Autodesk Fusion 360 part; units mm, degrees
(part 6 of 6)
extrude "Extrude3" cut sketch "Sketch2" along normal blind 1 contours L6 L7 L8 L9 L10 A2 | L11 L12 L13 L14 | L15 L16 L17 L18 L19 L20 | L21 L22 L23 L24 L25 A1 | L26 L27 L28 L29 | L30 L31 L32 L33 L34 A4 | L35 L36 L37 L38 L39 A3 | A0 | L40 L62 L64 L70 | L41 A7 L61 L63 L67 L73 | A5 L43 L48 L52 L55 L60 | A6 | L42 L46 L47 L54 L59 A8 | L44 L49 L53 L56 | L45 L50 L57 L66 L68 L71 | L51 L58 A9 L65 L69 L72 | L74 L96 L98 L104 | L75 A12 L95 L97 L101 L107 | A10 L77 L82 L86 L89 L94 | A11 | L76 L80 L81 L88 L93 A13 | L78 L83 L87 L90 | L79 L84 L91 L100 L102 L105 | L85 L92 A14 L99 L103 L106 | L108 L130 L132 L138 | L109 A17 L129 L131 L135 L141 | A15 L111 L116 L120 L123 L128 | A16 | L110 L114 L115 L122 L127 A18 | L112 L117 L121 L124 | L113 L118 L125 L134 L136 L139 | L119 L126 A19 L133 L137 L140 | L142 L164 L166 L172 | L143 A22 L163 L165 L169 L175 | A20 L145 L150 L154 L157 L162 | A21 | L144 L148 L149 L156 L161 A23 | L146 L151 L155 L158 | L147 L152 L159 L168 L170 L173 | L153 L160 A24 L167 L171 L174 | L176 L198 L200 L206 | L177 A27 L197 L199 L203 L209 | A25 L179 L184 L188 L191 L196 | A26 | L178 L182 L183 L190 L195 A28 | L180 L185 L189 L192 | L181 L186 L193 L202 L204 L207 | L187 L194 A29 L201 L205 L208 | L210 L232 L234 L240 | L211 A32 L231 L233 L237 L243 | A30 L213 L218 L222 L225 L230 | A31 | L212 L216 L217 L224 L229 A33 | L214 L219 L223 L226 | L215 L220 L227 L236 L238 L241 | L221 L228 A34 L235 L239 L242 | L244 L266 L268 L274 | L245 A37 L265 L267 L271 L277 | A35 L247 L252 L256 L259 L264 | A36 | L246 L250 L251 L258 L263 A38 | L248 L253 L257 L260 | L249 L254 L261 L270 L272 L275 | L255 L262 A39 L269 L273 L276 | L278 L300 L302 L308 | L279 A42 L299 L301 L305 L311 | A40 L281 L286 L290 L293 L298 | A41 | L280 L284 L285 L292 L297 A43 | L282 L287 L291 L294 | L283 L288 L295 L304 L306 L309 | L289 L296 A44 L303 L307 L310 | L312 L334 L336 L342 | L313 A47 L333 L335 L339 L345 | A45 L315 L320 L324 L327 L332 | A46 | L314 L318 L319 L326 L331 A48 | L316 L321 L325 L328 | L317 L322 L329 L338 L340 L343 | L323 L330 A49 L337 L341 L344 | L346 L368 L370 L376 | L347 A52 L367 L369 L373 L379 | A50 L349 L354 L358 L361 L366 | A51 | L348 L352 L353 L360 L365 A53 | L350 L355 L359 L362 | L351 L356 L363 L372 L374 L377 | L357 L364 A54 L371 L375 L378 | L380 L402 L404 L410 | L381 A57 L401 L403 L407 L413 | A55 L383 L388 L392 L395 L400 | A56 | L382 L386 L387 L394 L399 A58 | L384 L389 L393 L396 | L385 L390 L397 L406 L408 L411 | L391 L398 A59 L405 L409 L412 | L414 L436 L438 L444 | L415 A62 L435 L437 L441 L447 | A60 L417 L422 L426 L429 L434 | A61 | L416 L420 L421 L428 L433 A63 | L418 L423 L427 L430 | L419 L424 L431 L440 L442 L445 | L425 L432 A64 L439 L443 L446 | L448 L470 L472 L478 | L449 A67 L469 L471 L475 L481 | A65 L451 L456 L460 L463 L468 | A66 | L450 L454 L455 L462 L467 A68 | L452 L457 L461 L464 | L453 L458 L465 L474 L476 L479 | L459 L466 A69 L473 L477 L480 | L482 L504 L506 L512 | L483 A72 L503 L505 L509 L515 | A70 L485 L490 L494 L497 L502 | A71 | L484 L488 L489 L496 L501 A73 | L486 L491 L495 L498 | L487 L492 L499 L508 L510 L513 | L493 L500 A74 L507 L511 L514 | L516 L538 L540 L546 | L517 A77 L537 L539 L543 L549 | A75 L519 L524 L528 L531 L536 | A76 | L518 L522 L523 L530 L535 A78 | L520 L525 L529 L532 | L521 L526 L533 L542 L544 L547 | L527 L534 A79 L541 L545 L548 | L550 L572 L574 L580 | L551 A82 L571 L573 L577 L583 | A80 L553 L558 L562 L565 L570 | A81 | L552 L556 L557 L564 L569 A83 | L554 L559 L563 L566 | L555 L560 L567 L576 L578 L581 | L561 L568 A84 L575 L579 L582 | L584 L606 L608 L614 | L585 A87 L605 L607 L611 L617 | A85 L587 L592 L596 L599 L604 | A86 | L586 L590 L591 L598 L603 A88 | L588 L593 L597 L600 | L589 L594 L601 L610 L612 L615 | L595 L602 A89 L609 L613 L616 | L618 L640 L642 L648 | L619 A92 L639 L641 L645 L651 | A90 L621 L626 L630 L633 L638 | A91 | L620 L624 L625 L632 L637 A93 | L622 L627 L631 L634 | L623 L628 L635 L644 L646 L649 | L629 L636 A94 L643 L647 L650 | L652 L674 L676 L682 | L653 A97 L673 L675 L679 L685 | A95 L655 L660 L664 L667 L672 | A96 | L654 L658 L659 L666 L671 A98 | L656 L661 L665 L668 | L657 L662 L669 L678 L680 L683 | L663 L670 A99 L677 L681 L684 | L686 L708 L710 L716 | L687 A102 L707 L709 L713 L719 | A100 L689 L694 L698 L701 L706 | A101 | L688 L692 L693 L700 L705 A103 | L690 L695 L699 L702 | L691 L696 L703 L712 L714 L717 | L697 L704 A104 L711 L715 L718 | L720 L742 L744 L750 | L721 A107 L741 L743 L747 L753 | A105 L723 L728 L732 L735 L740 | A106 | L722 L726 L727 L734 L739 A108 | L724 L729 L733 L736 | L725 L730 L737 L746 L748 L751 | L731 L738 A109 L745 L749 L752 | L754 L776 L778 L784 | L755 A112 L775 L777 L781 L787 | A110 L757 L762 L766 L769 L774 | A111 | L756 L760 L761 L768 L773 A113 | L758 L763 L767 L770 | L759 L764 L771 L780 L782 L785 | L765 L772 A114 L779 L783 L786 | L788 L810 L812 L818 | L789 A117 L809 L811 L815 L821 | A115 L791 L796 L800 L803 L808 | A116 | L790 L794 L795 L802 L807 A118 | L792 L797 L801 L804 | L793 L798 L805 L814 L816 L819 | L799 L806 A119 L813 L817 L820 | L822 L844 L846 L852 | L823 A122 L843 L845 L849 L855 | A120 L825 L830 L834 L837 L842 | A121 | L824 L828 L829 L836 L841 A123 | L826 L831 L835 L838 | L827 L832 L839 L848 L850 L853 | L833 L840 A124 L847 L851 L854 | L856 L878 L880 L886 | L857 A127 L877 L879 L883 L889 | A125 L859 L864 L868 L871 L876 | A126 | L858 L862 L863 L870 L875 A128 | L860 L865 L869 L872 | L861 L866 L873 L882 L884 L887 | L867 L874 A129 L881 L885 L888 | L890 L912 L914 L920 | L891 A132 L911 L913 L917 L923 | A130 L893 L898 L902 L905 L910 | A131 | L892 L896 L897 L904 L909 A133 | L894 L899 L903 L906 | L895 L900 L907 L916 L918 L921 | L901 L908 A134 L915 L919 L922 | L924 L946 L948 L954 | L925 A137 L945 L947 L951 L957 | A135 L927 L932 L936 L939 L944 | A136 | L926 L930 L931 L938 L943 A138 | L928 L933 L937 L940 | L929 L934 L941 L950 L952 L955 | L935 L942 A139 L949 L953 L956 | L958 L980 L982 L988 | L959 A142 L979 L981 L985 L991 | A140 L961 L966 L970 L973 L978 | A141 | L960 L964 L965 L972 L977 A143 | L962 L967 L971 L974 | L963 L968 L975 L984 L986 L989 | L969 L976 A144 L983 L987 L990 | L992 L1014 L1016 L1022 | L993 A147 L1013 L1015 L1019 L1025 | A145 L995 L1000 L1004 L1007 L1012 | A146 | L994 L998 L999 L1006 L1011 A148 | L996 L1001 L1005 L1008 | L997 L1002 L1009 L1018 L1020 L1023 | L1003 L1010 A149 L1017 L1021 L1024 | L1026 L1048 L1050 L1056 | L1027 A152 L1047 L1049 L1053 L1059 | A150 L1029 L1034 L1038 L1041 L1046 | A151 | L1028 L1032 L1033 L1040 L1045 A153 | L1030 L1035 L1039 L1042 | L1031 L1036 L1043 L1052 L1054 L1057 | L1037 L1044 A154 L1051 L1055 L1058 | L1060 L1082 L1084 L1090 | L1061 A157 L1081 L1083 L1087 L1093 | A155 L1063 L1068 L1072 L1075 L1080 | A156 | L1062 L1066 L1067 L1074 L1079 A158 | L1064 L1069 L1073 L1076 | L1065 L1070 L1077 L1086 L1088 L1091 | L1071 L1078 A159 L1085 L1089 L1092
extrude "Extrude4" cut sketch "Sketch2" along normal blind 1 contours L1094 L1116 L1118 L1124 | L1095 A162 L1115 L1117 L1121 L1127 | A160 L1097 L1102 L1106 L1109 L1114 | A161 | L1096 L1100 L1101 L1108 L1113 A163 | L1098 L1103 L1107 L1110 | L1099 L1104 L1111 L1120 L1122 L1125 | L1105 L1112 A164 L1119 L1123 L1126 | L1128 L1150 L1152 L1158 | L1129 A167 L1149 L1151 L1155 L1161 | A165 L1131 L1136 L1140 L1143 L1148 | A166 | L1130 L1134 L1135 L1142 L1147 A168 | L1132 L1137 L1141 L1144 | L1133 L1138 L1145 L1154 L1156 L1159 | L1139 L1146 A169 L1153 L1157 L1160 | L1162 L1184 L1186 L1192 | L1163 A172 L1183 L1185 L1189 L1195 | A170 L1165 L1170 L1174 L1177 L1182 | A171 | L1164 L1168 L1169 L1176 L1181 A173 | L1166 L1171 L1175 L1178 | L1167 L1172 L1179 L1188 L1190 L1193 | L1173 L1180 A174 L1187 L1191 L1194 | L1196 L1218 L1220 L1226 | L1197 A177 L1217 L1219 L1223 L1229 | A175 L1199 L1204 L1208 L1211 L1216 | A176 | L1198 L1202 L1203 L1210 L1215 A178 | L1200 L1205 L1209 L1212 | L1201 L1206 L1213 L1222 L1224 L1227 | L1207 L1214 A179 L1221 L1225 L1228 | L1230 L1252 L1254 L1260 | L1231 A182 L1251 L1253 L1257 L1263 | A180 L1233 L1238 L1242 L1245 L1250 | A181 | L1232 L1236 L1237 L1244 L1249 A183 | L1234 L1239 L1243 L1246 | L1235 L1240 L1247 L1256 L1258 L1261 | L1241 L1248 A184 L1255 L1259 L1262 | L1264 L1286 L1288 L1294 | L1265 A187 L1285 L1287 L1291 L1297 | A185 L1267 L1272 L1276 L1279 L1284 | A186 | L1266 L1270 L1271 L1278 L1283 A188 | L1268 L1273 L1277 L1280 | L1269 L1274 L1281 L1290 L1292 L1295 | L1275 L1282 A189 L1289 L1293 L1296 | L1298 L1320 L1322 L1328 | L1299 A192 L1319 L1321 L1325 L1331 | A190 L1301 L1306 L1310 L1313 L1318 | A191 | L1300 L1304 L1305 L1312 L1317 A193 | L1302 L1307 L1311 L1314 | L1303 L1308 L1315 L1324 L1326 L1329 | L1309 L1316 A194 L1323 L1327 L1330 | L1332 L1354 L1356 L1362 | L1333 A197 L1353 L1355 L1359 L1365 | A195 L1335 L1340 L1344 L1347 L1352 | A196 | L1334 L1338 L1339 L1346 L1351 A198 | L1336 L1341 L1345 L1348 | L1337 L1342 L1349 L1358 L1360 L1363 | L1343 L1350 A199 L1357 L1361 L1364 | L1366 L1388 L1390 L1396 | L1367 A202 L1387 L1389 L1393 L1399 | A200 L1369 L1374 L1378 L1381 L1386 | A201 | L1368 L1372 L1373 L1380 L1385 A203 | L1370 L1375 L1379 L1382 | L1371 L1376 L1383 L1392 L1394 L1397 | L1377 L1384 A204 L1391 L1395 L1398 | L1400 L1422 L1424 L1430 | L1401 A207 L1421 L1423 L1427 L1433 | A205 L1403 L1408 L1412 L1415 L1420 | A206 | L1402 L1406 L1407 L1414 L1419 A208 | L1404 L1409 L1413 L1416 | L1405 L1410 L1417 L1426 L1428 L1431 | L1411 L1418 A209 L1425 L1429 L1432 | L1434 L1456 L1458 L1464 | L1435 A212 L1455 L1457 L1461 L1467 | A210 L1437 L1442 L1446 L1449 L1454 | A211 | L1436 L1440 L1441 L1448 L1453 A213 | L1438 L1443 L1447 L1450 | L1439 L1444 L1451 L1460 L1462 L1465 | L1445 L1452 A214 L1459 L1463 L1466 | L1468 L1490 L1492 L1498 | L1469 A217 L1489 L1491 L1495 L1501 | A215 L1471 L1476 L1480 L1483 L1488 | A216 | L1470 L1474 L1475 L1482 L1487 A218 | L1472 L1477 L1481 L1484 | L1473 L1478 L1485 L1494 L1496 L1499 | L1479 L1486 A219 L1493 L1497 L1500 | L1502 L1524 L1526 L1532 | L1503 A222 L1523 L1525 L1529 L1535 | A220 L1505 L1510 L1514 L1517 L1522 | A221 | L1504 L1508 L1509 L1516 L1521 A223 | L1506 L1511 L1515 L1518 | L1507 L1512 L1519 L1528 L1530 L1533 | L1513 L1520 A224 L1527 L1531 L1534 | L1536 L1558 L1560 L1566 | L1537 A227 L1557 L1559 L1563 L1569 | A225 L1539 L1544 L1548 L1551 L1556 | A226 | L1538 L1542 L1543 L1550 L1555 A228 | L1540 L1545 L1549 L1552 | L1541 L1546 L1553 L1562 L1564 L1567 | L1547 L1554 A229 L1561 L1565 L1568 | L1570 L1592 L1594 L1600 | L1571 A232 L1591 L1593 L1597 L1603 | A230 L1573 L1578 L1582 L1585 L1590 | A231 | L1572 L1576 L1577 L1584 L1589 A233 | L1574 L1579 L1583 L1586 | L1575 L1580 L1587 L1596 L1598 L1601 | L1581 L1588 A234 L1595 L1599 L1602 | L1604 L1626 L1628 L1634 | L1605 A237 L1625 L1627 L1631 L1637 | A235 L1607 L1612 L1616 L1619 L1624 | A236 | L1606 L1610 L1611 L1618 L1623 A238 | L1608 L1613 L1617 L1620 | L1609 L1614 L1621 L1630 L1632 L1635 | L1615 L1622 A239 L1629 L1633 L1636 | L1638 L1660 L1662 L1668 | L1639 A242 L1659 L1661 L1665 L1671 | A240 L1641 L1646 L1650 L1653 L1658 | A241 | L1640 L1644 L1645 L1652 L1657 A243 | L1642 L1647 L1651 L1654 | L1643 L1648 L1655 L1664 L1666 L1669 | L1649 L1656 A244 L1663 L1667 L1670 | L1672 L1694 L1696 L1702 | L1673 A247 L1693 L1695 L1699 L1705 | A245 L1675 L1680 L1684 L1687 L1692 | A246 | L1674 L1678 L1679 L1686 L1691 A248 | L1676 L1681 L1685 L1688 | L1677 L1682 L1689 L1698 L1700 L1703 | L1683 L1690 A249 L1697 L1701 L1704 | L1706 L1728 L1730 L1736 | L1707 A252 L1727 L1729 L1733 L1739 | A250 L1709 L1714 L1718 L1721 L1726 | A251 | L1708 L1712 L1713 L1720 L1725 A253 | L1710 L1715 L1719 L1722 | L1711 L1716 L1723 L1732 L1734 L1737 | L1717 L1724 A254 L1731 L1735 L1738 | L1740 L1762 L1764 L1770 | L1741 A257 L1761 L1763 L1767 L1773 | A255 L1743 L1748 L1752 L1755 L1760 | A256 | L1742 L1746 L1747 L1754 L1759 A258 | L1744 L1749 L1753 L1756 | L1745 L1750 L1757 L1766 L1768 L1771 | L1751 L1758 A259 L1765 L1769 L1772 | L1774 L1796 L1798 L1804 | L1775 A262 L1795 L1797 L1801 L1807 | A260 L1777 L1782 L1786 L1789 L1794 | A261 | L1776 L1780 L1781 L1788 L1793 A263 | L1778 L1783 L1787 L1790 | L1779 L1784 L1791 L1800 L1802 L1805 | L1785 L1792 A264 L1799 L1803 L1806 | L1808 L1830 L1832 L1838 | L1809 A267 L1829 L1831 L1835 L1841 | A265 L1811 L1816 L1820 L1823 L1828 | A266 | L1810 L1814 L1815 L1822 L1827 A268 | L1812 L1817 L1821 L1824 | L1813 L1818 L1825 L1834 L1836 L1839 | L1819 L1826 A269 L1833 L1837 L1840 | L1842 L1864 L1866 L1872 | L1843 A272 L1863 L1865 L1869 L1875 | A270 L1845 L1850 L1854 L1857 L1862 | A271 | L1844 L1848 L1849 L1856 L1861 A273 | L1846 L1851 L1855 L1858 | L1847 L1852 L1859 L1868 L1870 L1873 | L1853 L1860 A274 L1867 L1871 L1874 | L1876 L1898 L1900 L1906 | L1877 A277 L1897 L1899 L1903 L1909 | A275 L1879 L1884 L1888 L1891 L1896 | A276 | L1878 L1882 L1883 L1890 L1895 A278 | L1880 L1885 L1889 L1892 | L1881 L1886 L1893 L1902 L1904 L1907 | L1887 L1894 A279 L1901 L1905 L1908 | L1910 L1932 L1934 L1940 | L1911 A282 L1931 L1933 L1937 L1943 | A280 L1913 L1918 L1922 L1925 L1930 | A281 | L1912 L1916 L1917 L1924 L1929 A283 | L1914 L1919 L1923 L1926 | L1915 L1920 L1927 L1936 L1938 L1941 | L1921 L1928 A284 L1935 L1939 L1942 | L1944 L1966 L1968 L1974 | L1945 A287 L1965 L1967 L1971 L1977 | A285 L1947 L1952 L1956 L1959 L1964 | A286 | L1946 L1950 L1951 L1958 L1963 A288 | L1948 L1953 L1957 L1960 | L1949 L1954 L1961 L1970 L1972 L1975 | L1955 L1962 A289 L1969 L1973 L1976 | L1978 L2000 L2002 L2008 | L1979 A292 L1999 L2001 L2005 L2011 | A290 L1981 L1986 L1990 L1993 L1998 | A291 | L1980 L1984 L1985 L1992 L1997 A293 | L1982 L1987 L1991 L1994 | L1983 L1988 L1995 L2004 L2006 L2009 | L1989 L1996 A294 L2003 L2007 L2010 | L2012 L2034 L2036 L2042 | L2013 A297 L2033 L2035 L2039 L2045 | A295 L2015 L2020 L2024 L2027 L2032 | A296 | L2014 L2018 L2019 L2026 L2031 A298 | L2016 L2021 L2025 L2028 | L2017 L2022 L2029 L2038 L2040 L2043 | L2023 L2030 A299 L2037 L2041 L2044 | L2046 L2068 L2070 L2076 | L2047 A302 L2067 L2069 L2073 L2079 | A300 L2049 L2054 L2058 L2061 L2066 | A301 | L2048 L2052 L2053 L2060 L2065 A303 | L2050 L2055 L2059 L2062 | L2051 L2056 L2063 L2072 L2074 L2077 | L2057 L2064 A304 L2071 L2075 L2078 | L2080 L2102 L2104 L2110 | L2081 A307 L2101 L2103 L2107 L2113 | A305 L2083 L2088 L2092 L2095 L2100 | A306 | L2082 L2086 L2087 L2094 L2099 A308 | L2084 L2089 L2093 L2096 | L2085 L2090 L2097 L2106 L2108 L2111 | L2091 L2098 A309 L2105 L2109 L2112 | L2114 L2136 L2138 L2144 | L2115 A312 L2135 L2137 L2141 L2147 | A310 L2117 L2122 L2126 L2129 L2134 | A311 | L2116 L2120 L2121 L2128 L2133 A313 | L2118 L2123 L2127 L2130 | L2119 L2124 L2131 L2140 L2142 L2145 | L2125 L2132 A314 L2139 L2143 L2146 | L2148 L2170 L2172 L2178 | L2149 A317 L2169 L2171 L2175 L2181 | A315 L2151 L2156 L2160 L2163 L2168 | A316 | L2150 L2154 L2155 L2162 L2167 A318 | L2152 L2157 L2161 L2164 | L2153 L2158 L2165 L2174 L2176 L2179 | L2159 L2166 A319 L2173 L2177 L2180
extrude "Extrude5" cut sketch "Sketch2" along normal blind 1 contours L2182 L2204 L2206 L2212 | L2183 A322 L2203 L2205 L2209 L2215 | A320 L2185 L2190 L2194 L2197 L2202 | A321 | L2184 L2188 L2189 L2196 L2201 A323 | L2186 L2191 L2195 L2198 | L2187 L2192 L2199 L2208 L2210 L2213 | L2193 L2200 A324 L2207 L2211 L2214 | L2216 L2238 L2240 L2246 | L2217 A327 L2237 L2239 L2243 L2249 | A325 L2219 L2224 L2228 L2231 L2236 | A326 | L2218 L2222 L2223 L2230 L2235 A328 | L2220 L2225 L2229 L2232 | L2221 L2226 L2233 L2242 L2244 L2247 | L2227 L2234 A329 L2241 L2245 L2248 | L2250 L2272 L2274 L2280 | L2251 A332 L2271 L2273 L2277 L2283 | A330 L2253 L2258 L2262 L2265 L2270 | A331 | L2252 L2256 L2257 L2264 L2269 A333 | L2254 L2259 L2263 L2266 | L2255 L2260 L2267 L2276 L2278 L2281 | L2261 L2268 A334 L2275 L2279 L2282 | L2284 L2306 L2308 L2314 | L2285 A337 L2305 L2307 L2311 L2317 | A335 L2287 L2292 L2296 L2299 L2304 | A336 | L2286 L2290 L2291 L2298 L2303 A338 | L2288 L2293 L2297 L2300 | L2289 L2294 L2301 L2310 L2312 L2315 | L2295 L2302 A339 L2309 L2313 L2316 | L2318 L2340 L2342 L2348 | L2319 A342 L2339 L2341 L2345 L2351 | A340 L2321 L2326 L2330 L2333 L2338 | A341 | L2320 L2324 L2325 L2332 L2337 A343 | L2322 L2327 L2331 L2334 | L2323 L2328 L2335 L2344 L2346 L2349 | L2329 L2336 A344 L2343 L2347 L2350 | L2352 L2374 L2376 L2382 | L2353 A347 L2373 L2375 L2379 L2385 | A345 L2355 L2360 L2364 L2367 L2372 | A346 | L2354 L2358 L2359 L2366 L2371 A348 | L2356 L2361 L2365 L2368 | L2357 L2362 L2369 L2378 L2380 L2383 | L2363 L2370 A349 L2377 L2381 L2384 | L2386 L2408 L2410 L2416 | L2387 A352 L2407 L2409 L2413 L2419 | A350 L2389 L2394 L2398 L2401 L2406 | A351 | L2388 L2392 L2393 L2400 L2405 A353 | L2390 L2395 L2399 L2402 | L2391 L2396 L2403 L2412 L2414 L2417 | L2397 L2404 A354 L2411 L2415 L2418 | L2420 L2442 L2444 L2450 | L2421 A357 L2441 L2443 L2447 L2453 | A355 L2423 L2428 L2432 L2435 L2440 | A356 | L2422 L2426 L2427 L2434 L2439 A358 | L2424 L2429 L2433 L2436 | L2425 L2430 L2437 L2446 L2448 L2451 | L2431 L2438 A359 L2445 L2449 L2452 | L2454 L2476 L2478 L2484 | L2455 A362 L2475 L2477 L2481 L2487 | A360 L2457 L2462 L2466 L2469 L2474 | A361 | L2456 L2460 L2461 L2468 L2473 A363 | L2458 L2463 L2467 L2470 | L2459 L2464 L2471 L2480 L2482 L2485 | L2465 L2472 A364 L2479 L2483 L2486 | L2488 L2510 L2512 L2518 | L2489 A367 L2509 L2511 L2515 L2521 | A365 L2491 L2496 L2500 L2503 L2508 | A366 | L2490 L2494 L2495 L2502 L2507 A368 | L2492 L2497 L2501 L2504 | L2493 L2498 L2505 L2514 L2516 L2519 | L2499 L2506 A369 L2513 L2517 L2520 | L2522 L2544 L2546 L2552 | L2523 A372 L2543 L2545 L2549 L2555 | A370 L2525 L2530 L2534 L2537 L2542 | A371 | L2524 L2528 L2529 L2536 L2541 A373 | L2526 L2531 L2535 L2538 | L2527 L2532 L2539 L2548 L2550 L2553 | L2533 L2540 A374 L2547 L2551 L2554 | L2556 L2578 L2580 L2586 | L2557 A377 L2577 L2579 L2583 L2589 | A375 L2559 L2564 L2568 L2571 L2576 | A376 | L2558 L2562 L2563 L2570 L2575 A378 | L2560 L2565 L2569 L2572 | L2561 L2566 L2573 L2582 L2584 L2587 | L2567 L2574 A379 L2581 L2585 L2588 | L2590 L2612 L2614 L2620 | L2591 A382 L2611 L2613 L2617 L2623 | A380 L2593 L2598 L2602 L2605 L2610 | A381 | L2592 L2596 L2597 L2604 L2609 A383 | L2594 L2599 L2603 L2606 | L2595 L2600 L2607 L2616 L2618 L2621 | L2601 L2608 A384 L2615 L2619 L2622 | L2624 L2646 L2648 L2654 | L2625 A387 L2645 L2647 L2651 L2657 | A385 L2627 L2632 L2636 L2639 L2644 | A386 | L2626 L2630 L2631 L2638 L2643 A388 | L2628 L2633 L2637 L2640 | L2629 L2634 L2641 L2650 L2652 L2655 | L2635 L2642 A389 L2649 L2653 L2656 | L2658 L2680 L2682 L2688 | L2659 A392 L2679 L2681 L2685 L2691 | A390 L2661 L2666 L2670 L2673 L2678 | A391 | L2660 L2664 L2665 L2672 L2677 A393 | L2662 L2667 L2671 L2674 | L2663 L2668 L2675 L2684 L2686 L2689 | L2669 L2676 A394 L2683 L2687 L2690 | L2692 L2714 L2716 L2722 | L2693 A397 L2713 L2715 L2719 L2725 | A395 L2695 L2700 L2704 L2707 L2712 | A396 | L2694 L2698 L2699 L2706 L2711 A398 | L2696 L2701 L2705 L2708 | L2697 L2702 L2709 L2718 L2720 L2723 | L2703 L2710 A399 L2717 L2721 L2724 | L2726 L2748 L2750 L2756 | L2727 A402 L2747 L2749 L2753 L2759 | A400 L2729 L2734 L2738 L2741 L2746 | A401 | L2728 L2732 L2733 L2740 L2745 A403 | L2730 L2735 L2739 L2742 | L2731 L2736 L2743 L2752 L2754 L2757 | L2737 L2744 A404 L2751 L2755 L2758 | L2760 L2782 L2784 L2790 | L2761 A407 L2781 L2783 L2787 L2793 | A405 L2763 L2768 L2772 L2775 L2780 | A406 | L2762 L2766 L2767 L2774 L2779 A408 | L2764 L2769 L2773 L2776 | L2765 L2770 L2777 L2786 L2788 L2791 | L2771 L2778 A409 L2785 L2789 L2792 | L2794 L2816 L2818 L2824 | L2795 A412 L2815 L2817 L2821 L2827 | A410 L2797 L2802 L2806 L2809 L2814 | A411 | L2796 L2800 L2801 L2808 L2813 A413 | L2798 L2803 L2807 L2810 | L2799 L2804 L2811 L2820 L2822 L2825 | L2805 L2812 A414 L2819 L2823 L2826 | L2828 L2850 L2852 L2858 | L2829 A417 L2849 L2851 L2855 L2861 | A415 L2831 L2836 L2840 L2843 L2848 | A416 | L2830 L2834 L2835 L2842 L2847 A418 | L2832 L2837 L2841 L2844 | L2833 L2838 L2845 L2854 L2856 L2859 | L2839 L2846 A419 L2853 L2857 L2860 | L2862 L2884 L2886 L2892 | L2863 A422 L2883 L2885 L2889 L2895 | A420 L2865 L2870 L2874 L2877 L2882 | A421 | L2864 L2868 L2869 L2876 L2881 A423 | L2866 L2871 L2875 L2878 | L2867 L2872 L2879 L2888 L2890 L2893 | L2873 L2880 A424 L2887 L2891 L2894 | L2896 L2918 L2920 L2926 | L2897 A427 L2917 L2919 L2923 L2929 | A425 L2899 L2904 L2908 L2911 L2916 | A426 | L2898 L2902 L2903 L2910 L2915 A428 | L2900 L2905 L2909 L2912 | L2901 L2906 L2913 L2922 L2924 L2927 | L2907 L2914 A429 L2921 L2925 L2928 | L2930 L2952 L2954 L2960 | L2931 A432 L2951 L2953 L2957 L2963 | A430 L2933 L2938 L2942 L2945 L2950 | A431 | L2932 L2936 L2937 L2944 L2949 A433 | L2934 L2939 L2943 L2946 | L2935 L2940 L2947 L2956 L2958 L2961 | L2941 L2948 A434 L2955 L2959 L2962 | L2964 L2986 L2988 L2994 | L2965 A437 L2985 L2987 L2991 L2997 | A435 L2967 L2972 L2976 L2979 L2984 | A436 | L2966 L2970 L2971 L2978 L2983 A438 | L2968 L2973 L2977 L2980 | L2969 L2974 L2981 L2990 L2992 L2995 | L2975 L2982 A439 L2989 L2993 L2996 | L2998 L3020 L3022 L3028 | L2999 A442 L3019 L3021 L3025 L3031 | A440 L3001 L3006 L3010 L3013 L3018 | A441 | L3000 L3004 L3005 L3012 L3017 A443 | L3002 L3007 L3011 L3014 | L3003 L3008 L3015 L3024 L3026 L3029 | L3009 L3016 A444 L3023 L3027 L3030 | L3032 L3054 L3056 L3062 | L3033 A447 L3053 L3055 L3059 L3065 | A445 L3035 L3040 L3044 L3047 L3052 | A446 | L3034 L3038 L3039 L3046 L3051 A448 | L3036 L3041 L3045 L3048 | L3037 L3042 L3049 L3058 L3060 L3063 | L3043 L3050 A449 L3057 L3061 L3064 | L3066 L3088 L3090 L3096 | L3067 A452 L3087 L3089 L3093 L3099 | A450 L3069 L3074 L3078 L3081 L3086 | A451 | L3068 L3072 L3073 L3080 L3085 A453 | L3070 L3075 L3079 L3082 | L3071 L3076 L3083 L3092 L3094 L3097 | L3077 L3084 A454 L3091 L3095 L3098 | L3100 L3122 L3124 L3130 | L3101 A457 L3121 L3123 L3127 L3133 | A455 L3103 L3108 L3112 L3115 L3120 | A456 | L3102 L3106 L3107 L3114 L3119 A458 | L3104 L3109 L3113 L3116 | L3105 L3110 L3117 L3126 L3128 L3131 | L3111 L3118 A459 L3125 L3129 L3132 | L3134 L3156 L3158 L3164 | L3135 A462 L3155 L3157 L3161 L3167 | A460 L3137 L3142 L3146 L3149 L3154 | A461 | L3136 L3140 L3141 L3148 L3153 A463 | L3138 L3143 L3147 L3150 | L3139 L3144 L3151 L3160 L3162 L3165 | L3145 L3152 A464 L3159 L3163 L3166 | L3168 L3190 L3192 L3198 | L3169 A467 L3189 L3191 L3195 L3201 | A465 L3171 L3176 L3180 L3183 L3188 | A466 | L3170 L3174 L3175 L3182 L3187 A468 | L3172 L3177 L3181 L3184 | L3173 L3178 L3185 L3194 L3196 L3199 | L3179 L3186 A469 L3193 L3197 L3200 | L3202 L3224 L3226 L3232 | L3203 A472 L3223 L3225 L3229 L3235 | A470 L3205 L3210 L3214 L3217 L3222 | A471 | L3204 L3208 L3209 L3216 L3221 A473 | L3206 L3211 L3215 L3218 | L3207 L3212 L3219 L3228 L3230 L3233 | L3213 L3220 A474 L3227 L3231 L3234 | L3236 L3258 L3260 L3266 | L3237 A477 L3257 L3259 L3263 L3269 | A475 L3239 L3244 L3248 L3251 L3256 | A476 | L3238 L3242 L3243 L3250 L3255 A478 | L3240 L3245 L3249 L3252 | L3241 L3246 L3253 L3262 L3264 L3267 | L3247 L3254 A479 L3261 L3265 L3268
extrude "Extrude2" [suppressed]
equation "d1 = ( ( 610 / 3 ) * 1 mm )"
equation "d2 = ( 459 / 4 ) * 1 mm"
equation "d6 = d5 / 16"
equation "d7 = d8 / 6"
equation "d10 = d15 + d9 / 2"
equation "d26 = d19 / 2"
equation "d44 = d43 / 2 - 0.1 mm"

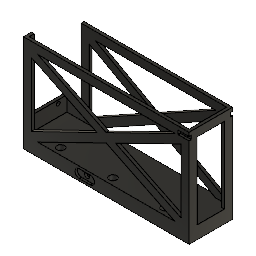
design "Power Supply Case"
Autodesk Fusion 360 part; units mm, degrees
sketch "Sketch1" plane through (0, 0, 0) normal (0, 0, 1) x (1, 0, 0)
  line L0 (0, 0) -> (214.5, 0)
  line L1 (214.5, 0) -> (214.5, 50.5)
  line L2 (214.5, 50.5) -> (0, 50.5)
  line L3 (0, 50.5) -> (0, 0)
  line L4 (-4, -4) -> (218.5, -4)
  line L5 (218.5, -4) -> (218.5, 54.5)
  line L6 (218.5, 54.5) -> (-4, 54.5)
  line L7 (-4, 54.5) -> (-4, -4)
  line L8 (7, 0) -> (7, -4)
  line L9 (0, 7) -> (-4, 7)
  line L10 (207.5, 0) -> (207.5, -4)
  line L11 (214.5, 7) -> (218.5, 7)
  line L12 (207.5, 54.5) -> (207.5, 50.5)
  line L13 (214.5, 43.5) -> (218.5, 43.5)
  line L14 (19, 50.5) -> (19, 54.5)
  line L15 (30, 50.5) -> (30, 54.5)
  line L16 (0, 36.5) -> (-4, 36.5)
  line L17 (0, 41.5) -> (-4, 41.5)
  point P0 (37.25, 5)
  point P1 (107.25, 5)
  point P2 (177.25, 5)
  dimension "d1" = 4
  dimension "d2" = 4
  dimension "d3" = 4
  dimension "d4" = 4
  dimension "d5" = 50.5
  dimension "d6" = 214.5
  dimension "d7" = 70
  dimension "d8" = 70
  dimension "d9" = 37.25
  dimension "d27" = 7
  dimension "d28" = 7
  dimension "d29" = 7
  dimension "d30" = 7
  dimension "d31" = 7
  dimension "d32" = 7
  dimension "d53" = 11
  dimension "d54" = 19
  dimension "d61" = 5
  dimension "d62" = 5
  dimension "d63" = 5
  dimension "d66" = 14
  dimension "d67" = 9
  constraint horizontal L0
  constraint vertical L1
  constraint horizontal L2
  constraint vertical L3
  constraint coincident L0.start L3.end
  constraint horizontal L4
  constraint vertical L5
  constraint horizontal L6
  constraint vertical L7
  constraint coincident L0 L8.start
  constraint coincident L4 L8.end
  constraint perpendicular L4 L8
  constraint coincident L3 L9.start
  constraint perpendicular L3 L9
  constraint coincident L0 L10.start
  constraint coincident L4 L10.end
  constraint perpendicular L4 L10
  constraint coincident L1 L11.start
  constraint coincident L5 L11.end
  constraint perpendicular L5 L11
  constraint coincident L6 L12.start
  constraint coincident L2 L12.end
  constraint perpendicular L2 L12
  constraint coincident L1 L13.start
  constraint coincident L5 L13.end
  constraint perpendicular L5 L13
  constraint coincident L7 L9.end
  constraint coincident L2 L14.start
  constraint coincident L6 L14.end
  constraint perpendicular L6 L14
  constraint coincident L2 L15.start
  constraint coincident L6 L15.end
  constraint perpendicular L2 L15
  constraint coincident L3 L16.start
  constraint coincident L7 L16.end
  constraint perpendicular L7 L16
  constraint coincident L3 L17.start
  constraint coincident L7 L17.end
  constraint perpendicular L7 L17
  measures "d1" distance of L0 L4
  measures "d2" distance of L3 L7
  measures "d3" distance of L1 L5
  measures "d4" distance of L2 L6
  measures "d5" distance of L0.start L2.end
  measures "d6" distance of L0.start L0.end
  measures "d7" distance of P0 P1
  measures "d8" distance of P1 P2
  measures "d9" horizontal distance of L0.start P0
  measures "d27" distance of L0.start L8
  measures "d28" distance of L0.start L9
  measures "d29" distance of L0.end L10
  measures "d30" distance of L0.end L11
  measures "d31" distance of L1.end L13
  measures "d32" distance of L1.end L12
  measures "d53" distance of L14 L15
  measures "d54" distance of L2.end L14
  measures "d61" distance of L0 P0
  measures "d62" distance of L0 P1
  measures "d63" distance of L0 P2
  measures "d66" distance of L2 L16
  measures "d67" distance of L2 L17
extrude "Extrude1" add sketch "Sketch1" against normal blind 17.5
hole "Hole1" at (37.25, 5, 0) at (107.25, 5, 0) at (177.25, 5, 0) direction (0, 0, -1) diameter 6.5 end up to surface (17.5 mm away) counterbore diameter 10 counterbore depth 6.5
extrude "Extrude3" add sketch "Sketch1" along normal blind 113 contours L0 L3 L4 L7 L8 L9 | L0 L4 L8 L10 | L0 L1 L4 L5 L10 L11 | L1 L5 L11 L13 | L1 L2 L5 L6 L12 L13 | L2 L6 L14 L15 | L2 L6 L12 L15
extrude "Extrude4" cut sketch "Sketch1" along normal blind 102 contours L0 L4 L8 L10 | L1 L5 L11 L13 | L2 L6 L12 L15
extrude "Extrude9" add sketch "Sketch1" along normal blind 20 contours L3 L7 L9 L16 | L3 L7 L16 L17 | L2 L3 L6 L7 L14 L17
extrude "Extrude10" cut sketch "Sketch1" along normal blind 18 contours L3 L7 L16 L17
extrude "Extrude13" add sketch "Sketch1" along normal blind 13 contours L3 L7 L16 L17
fillet "Fillet1" radius 2.5 4 edges at (-2, 41.5, 13) (-2, 36.5, 13) (-2, 36.5, 18) (-2, 41.5, 18)
sketch "Sketch2" plane through (0, -4, 0) normal (0, -1, 0) x (1, 0, 0)
  line L0 (7, 0) -> (7, 102)
  line L1 (7, 102) -> (207.5, 102)
  line L2 (207.5, 102) -> (207.5, 0)
  line L3 (207.5, 0) -> (7, 0)
  line L4 (-4, 113) -> (-4, -17.5)
  line L5 (-4, -17.5) -> (218.5, -17.5)
  line L6 (218.5, -17.5) -> (218.5, 113)
  line L7 (218.5, 113) -> (-4, 113)
  line L8 (7, 93.7736) -> (199.2736, 0)
  line L9 (15.2264, 102) -> (207.5, 8.2264)
  line L10 (199.2736, 102) -> (7, 8.2264)
  line L11 (207.5, 93.7736) -> (15.2264, 0)
  line L12 (-4, 0) -> (218.5, 0)
  line L13 (30, 0) -> (30, 102)
  line L14 (7, 93.7736) -> (7, 102)
  line L15 (7, 102) -> (15.2264, 102)
  line L16 (7, 8.2264) -> (7, 0)
  line L17 (15.2264, 0) -> (7, 0)
  line L18 (86, -3.125) -> (71, -3.125)
  line L19 (86, -8.75) -> (71, -8.75) construction
  line L20 (71, -14.375) -> (86, -14.375)
  arc A0 (86, -14.375) -> (86, -3.125) centre (86, -8.75) ccw
  arc A1 (71, -3.125) -> (71, -14.375) centre (71, -8.75) ccw
  point P0 (94.7031, 51)
  point P1 (7, 0)
  point P2 (207.5, 0)
  point P3 (78.5, -8.75)
  dimension "d37" = 11
  dimension "d38" = 11
  dimension "d47" = 51
  dimension "d48" = 102
  dimension "d89" = 5.625
  dimension "d90" = 15
  dimension "d91" = 17.5
  dimension "d92" = 8.75
  dimension "d93" = 140
  constraint coincident L3 L8.end
  constraint coincident L3 L11.end
  constraint parallel L10 L11
  constraint parallel L8 L9
  constraint coincident L10 P0
  constraint coincident L8 P0
  constraint coincident L2 L9.end
  constraint coincident L2 L11.start
  constraint coincident L1 L10.start
  constraint coincident L1 L9.start
  constraint equal L8 L9
  constraint equal L14 L15
  constraint equal L16 L17
  constraint coincident L0 L10.end
  constraint coincident P1 L0.start
  constraint coincident L0 L8.start
  constraint coincident L0.end L1.start
  constraint tangent L18 A1
  constraint tangent L20 A1
  constraint parallel L18 L20
  constraint tangent L20 A0
  constraint tangent L18 A0
  constraint horizontal L19
  constraint midpoint P3 L19
  measures "d37" distance of L8 L9
  measures "d38" distance of L10 L11
  measures "d47" distance of P0 L12
  measures "d48" distance of L0.start L0.end
  measures "d89" radius of A1
  measures "d90" distance of L19.start L19.end
  measures "d91" distance of L5 L12
  measures "d92" distance of L12 P3
  measures "d93" distance of L6 P3
extrude "Extrude7" add sketch "Sketch2" against normal blind 4 contours L0 L3 L10 L11 L12 L13 L16 L17 | L0 L1 L8 L9 L13 L14 L15 | L8 L10 L11 L13 | L8 L9 L10 L13 | L8 L9 L10 L11 | L2 L3 L8 L9 L11 L12 | L1 L2 L9 L10 L11
sketch "Sketch3" plane through (0, 54.5, 0) normal (0, 1, 0) x (-1, 0, 0)
  line L0 (-19, 113) -> (-218.5, 113)
  line L1 (-218.5, 113) -> (-218.5, -17.5)
  line L2 (-218.5, -17.5) -> (4, -17.5)
  line L3 (4, -17.5) -> (4, 20)
  line L4 (-30, 102) -> (-30, 0)
  line L5 (-30, 0) -> (-207.5, 0)
  line L6 (-207.5, 0) -> (-207.5, 102)
  line L7 (-207.5, 102) -> (-30, 102)
  line L8 (-207.5, 93.9084) -> (-38.0916, 0)
  line L9 (-30, 8.0916) -> (-199.4084, 102)
  line L10 (-199.4084, 102) -> (-207.5, 102)
  line L11 (-207.5, 93.9084) -> (-207.5, 102)
  line L12 (-207.5, 0) -> (-207.5, 8.0916)
  line L13 (-207.5, 8.0916) -> (-38.0916, 102)
  line L14 (-207.5, 0) -> (-199.4084, 0)
  line L15 (-199.4084, 0) -> (-30, 93.9084)
  line L16 (-19, 20) -> (-19, 113)
  line L17 (4, 20) -> (-19, 20)
  point P0 (-130.0943, 51)
  point P1 (-78.5, -8.75)
  dimension "d55" = 11
  dimension "d56" = 11
  dimension "d57" = 102
  dimension "d58" = 51
  dimension "d79" = 17.5
  dimension "d80" = 8.75
  dimension "d82" = 140
  constraint coincident L6 L8.start
  constraint coincident L5 L8.end
  constraint coincident L4 L9.start
  constraint coincident L7 L9.end
  constraint coincident L6.end L7.start
  constraint coincident L5.end L6.start
  constraint coincident L6 L12.end
  constraint perpendicular L5 L12
  constraint coincident L7 L13.end
  constraint coincident L5 L6.start
  constraint coincident L5 L14.end
  constraint coincident L4 L15.end
  constraint parallel L13 L15
  constraint parallel L8 L9
  constraint equal L8 L9
  constraint equal L10 L11
  constraint equal L12 L14
  constraint equal L13 L15
  constraint coincident L13 P0
  constraint coincident L8 P0
  measures "d55" distance of L8 L9
  measures "d56" distance of L13 L15
  measures "d57" distance of L5.end L6.end
  measures "d58" distance of L5 P0
  measures "d79" distance of L2 L5
  measures "d80" distance of L5 P1
  measures "d82" distance of L1 P1
extrude "Extrude8" add sketch "Sketch3" against normal up to surface (4 mm away) contours L4 L7 L9 L13 L15 | L4 L5 L8 L9 L15 | L8 L9 L13 L15 | L6 L7 L8 L9 L10 L11 L13 | L5 L6 L8 L12 L13 L14 L15
sketch "Sketch4" plane through (218.5, 0, 0) normal (1, 0, 0) x (0, 1, 0)
  line L0 (7, 0) -> (7, 102)
  line L1 (7, 102) -> (43.5, 102)
  line L2 (43.5, 102) -> (43.5, 0)
  line L3 (43.5, 0) -> (7, 0)
  line L4 (-4, 113) -> (-4, -17.5)
  line L5 (-4, -17.5) -> (54.5, -17.5)
  line L6 (54.5, -17.5) -> (54.5, 113)
  line L7 (54.5, 113) -> (-4, 113)
  line L8 (-4, 108) -> (-1, 108)
  line L9 (-1, 108) -> (-1, 103)
  line L10 (-1, 103) -> (-4, 103)
  line L11 (-4, 103) -> (-4, 108)
  line L12 (54.5, 108) -> (51.5, 108)
  line L13 (51.5, 108) -> (51.5, 103)
  line L14 (51.5, 103) -> (54.5, 103)
  line L15 (54.5, 103) -> (54.5, 108)
  dimension "d74" = 5
  dimension "d75" = 5
  dimension "d76" = 3
  constraint horizontal L8
  constraint vertical L9
  constraint horizontal L10
  constraint vertical L11
  constraint horizontal L12
  constraint vertical L13
  constraint horizontal L14
  constraint vertical L15
  constraint collinear L4 L11
  constraint collinear L6 L15
  constraint equal L9 L13
  constraint equal L8 L12
  constraint collinear L8 L12
  measures "d74" distance of L7 L8
  measures "d75" distance of L8.end L9.end
  measures "d76" distance of L9.end L10.end
extrude "Extrude11" cut sketch "Sketch4" against normal blind 15 contours L4 L8 L9 L10 L11 | L6 L12 L13 L14 L15
hole "Hole2" at (78.5, 54.5, -8.75) direction (0, -1, 0) diameter 6.5 end up to surface (58.5 mm away) counterbore diameter 10 counterbore depth 52.5
extrude "Extrude12" cut sketch "Sketch2" against normal blind 3 contours L18 L20 A0 A1
equation "d2 = d1"
equation "d3 = d1"
equation "d4 = d1"
equation "d8 = d7"
equation "d9 = ( d6 - d7 * 2 ) / 2"
equation "d28 = d27"
equation "d29 = d27"
equation "d30 = d27"
equation "d31 = d27"
equation "d32 = d27"
equation "d35 = 113 mm - 11 mm"
equation "d47 = d48 / 2"
equation "d58 = d57 / 2"
equation "d62 = d61"
equation "d63 = d61"
equation "d80 = d79 / 2"
equation "d86 = 58.5 mm - 6 mm"
equation "d92 = ( 17.5 / 2 ) * 1 mm"
